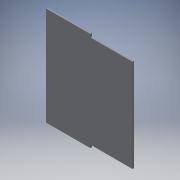
# Autodesk Inventor part: Dach2
Saved by Autodesk Inventor 2019 (Build 230136000, 136)
## iProperties
Created: 2023-01-16
Part Number: Dach2
Material: Ogólny
Document SubType Name: Modeling
Designer: Michał
Density: 1 g/cm^3
Appearance: Domyślna
Author: Michał
Autodesk Inventor part; units mm, degrees
ref_plane "YZ Plane" through (0, 0, 0) normal (1, 0, 0) x (0, 1, 0)
ref_plane "XZ Plane" through (0, 0, 0) normal (0, 1, 0) x (-1, 0, 0)
ref_plane "XY Plane" through (0, 0, 0) normal (0, 0, 1) x (1, 0, 0)
sketch "Szkic1" plane through (0, 0, 0) normal (0, 0, 1) x (1, 0, 0)
  line L0 (-30.3153, -10.76) -> (-97.6449, -10.76) construction
  line L1 (-30.3153, -10.76) -> (-97.6449, -10.76) construction
  line L2 (-101.109, 124.5875) -> (-101.109, -11.5875) construction
  line L3 (-30.3153, 123.76) -> (-97.6449, 123.76) construction
  line L4 (16.507, 124.589) -> (16.507, -11.589) construction
  line L5 (-40.75, -6.5) -> (16.507, -6.5) construction
  line L6 (-40.75, 119.5) -> (16.507, 119.5) construction
  line L7 (-100.909, 123.56) -> (-40.75, 123.56)
  line L8 (-40.75, 123.56) -> (-40.75, -10.56)
  line L9 (-40.75, -10.56) -> (-100.909, -10.56)
  line L10 (-100.909, -10.56) -> (-100.909, 123.56)
  line L11 (-40.75, 119.5) -> (16.307, 119.5)
  line L12 (16.307, 119.5) -> (16.307, -6.5)
  line L13 (16.307, -6.5) -> (-40.75, -6.5)
  line L14 (-40.75, -6.5) -> (-40.75, 119.5)
  line L15 (-100.909, 56.5) -> (-101.109, 56.5) construction
  line L16 (16.307, 56.5) -> (16.507, 56.5) construction
  line L17 (-70.8295, -10.56) -> (-70.8295, -10.76) construction
  line L18 (-70.8295, 123.56) -> (-70.8295, 123.76) construction
  line L19 (-89.609, 108.26) -> (-100.609, 108.26)
  line L20 (-89.609, 115.26) -> (-89.609, 108.26)
  line L21 (-100.609, 115.26) -> (-89.609, 115.26)
  line L22 (-100.609, 108.26) -> (-100.609, 115.26)
  line L23 (-100.609, 115.26) -> (-100.909, 115.26)
  line L24 (-100.609, 108.26) -> (-100.909, 108.26)
  line L25 (-87.109, 6.24) -> (-99.109, 6.24) projected
  line L26 (-99.109, -2.76) -> (-99.109, 6.24) projected
  line L27 (-87.109, -2.76) -> (-99.109, -2.76) projected
  line L28 (-87.109, 6.24) -> (-87.109, -2.76) projected
  line L29 (-75.109, 13.24) -> (-75.109, 6.24)
  line L30 (-75.109, 6.24) -> (-86.109, 6.24)
  line L31 (-86.109, 6.24) -> (-86.109, 13.24)
  line L32 (-86.109, 13.24) -> (-75.109, 13.24)
  line L33 (-85.609, 5.24) -> (-75.109, 5.24)
  line L34 (-75.109, 5.24) -> (-75.109, -9.76)
  line L35 (-75.109, -9.76) -> (-85.609, -9.76)
  line L36 (-85.609, -9.76) -> (-85.609, 5.24)
  line L37 (-76.109, -9.06) -> (-84.609, -9.06) construction
  line L38 (-84.609, -9.06) -> (-84.609, 4.54) construction
  line L39 (-84.609, 4.54) -> (-76.109, 4.54) construction
  line L40 (-76.109, 4.54) -> (-76.109, -9.06) construction
  line L41 (-75.109, 5.24) -> (-75.109, -9.76) construction
  line L42 (-85.609, 5.24) -> (-75.109, 5.24) construction
  line L43 (-85.609, -9.76) -> (-85.609, 5.24) construction
  line L44 (-75.109, -9.76) -> (-85.609, -9.76) construction
  line L45 (-75.109, -2.26) -> (-75.109, -2.26) construction
  line L46 (-75.109, -9.76) -> (-85.609, -9.76)
  line L47 (-85.609, -9.76) -> (-85.609, -10.56)
  line L48 (-85.609, -10.56) -> (-75.109, -10.56)
  line L49 (-75.109, -10.56) -> (-75.109, -9.76)
  point P0 (0, 0)
  point P1 (-40.75, 56.5)
  dimension "d0" = 0.2
  constraints: 62 end point, 10 midpoint, 10 perpendicular, 8 horizontal, 8 parallel, 7 collinear, 7 point on line, 4 vertical, 2 equal length, 8 other
  measures "d0" distance between parallel lines of L4 L12
ref_plane "Płaszczyzna konstrukcyjna1" through (16.507, -11.589, 2) normal (0, 0, 1) x (1, 0, 0)
extrude "Wyciągnięcie proste3" add sketch "Szkic1" along normal blind 2 contours L7 L8 L9 L49 L34 L33 L36 L47 L10 L24 L19 L20 L21 L23 | L11 L12 L13 L8
sketch "Szkic2" plane through (-100.909, 123.56, 2) normal (0, 0, 1) x (1, 0, 0)
  line L0 (98.216, -22.2759) -> (98.216, -111.8441) construction
  line L1 (98.216, -111.8441) -> (83.8317, -111.8441) construction
  line L2 (83.8317, -111.8441) -> (83.8317, -22.2759) construction
  line L3 (83.8317, -22.2759) -> (98.216, -22.2759) construction
  line L4 (81.8317, -22.2759) -> (81.8317, -80.9218) construction
  line L5 (81.8317, -80.9218) -> (73.6071, -80.9218) construction
  line L6 (73.6071, -80.9218) -> (73.6071, -22.2759) construction
  line L7 (73.6071, -22.2759) -> (81.8317, -22.2759) construction
  line L8 (35.5742, -109.2952) -> (35.5742, -118.3334) construction
  line L9 (35.5742, -118.3334) -> (29.6072, -118.3334) construction
  line L10 (29.6072, -118.3334) -> (29.6072, -109.2952) construction
  line L11 (29.6072, -109.2952) -> (35.5742, -109.2952) construction
  line L12 (36.1418, -121.3134) -> (36.1418, -131.569) construction
  line L13 (36.1418, -131.569) -> (29.1418, -131.569) construction
  line L14 (29.1418, -131.569) -> (29.1418, -121.3134) construction
  line L15 (29.1418, -121.3134) -> (36.1418, -121.3134) construction
  line L16 (21.349, -9.0957) -> (21.349, -16.2294) construction
  line L17 (21.349, -16.2294) -> (14.3259, -16.2294) construction
  line L18 (14.3259, -16.2294) -> (14.3259, -9.0957) construction
  line L19 (14.3259, -9.0957) -> (21.349, -9.0957) construction
  line L20 (13.8, -117.32) -> (13.8, -126.32) construction
  line L21 (13.8, -126.32) -> (1.8, -126.32) construction
  line L22 (1.8, -126.32) -> (1.8, -117.32) construction
  line L23 (1.8, -117.32) -> (13.8, -117.32) construction
  line L24 (25.8, -117.32) -> (14.8, -117.32) construction
  line L25 (14.8, -117.32) -> (14.8, -110.32) construction
  line L26 (14.8, -110.32) -> (25.8, -110.32) construction
  line L27 (25.8, -110.32) -> (25.8, -117.32) construction
  line L28 (60.159, -130.06) -> (117.216, -130.06) construction
  line L29 (117.216, -130.06) -> (117.216, -4.06) construction
  line L30 (117.216, -4.06) -> (60.159, -4.06) construction
  line L31 (60.159, -4.06) -> (60.159, 0) construction
  line L32 (60.159, 0) -> (0, 0) construction
  line L33 (0, 0) -> (0, -8.3) construction
  line L34 (0, -8.3) -> (11.3, -8.3) construction
  line L35 (11.3, -8.3) -> (11.3, -15.3) construction
  line L36 (11.3, -15.3) -> (0, -15.3) construction
  line L37 (0, -15.3) -> (0, -134.12) construction
  line L38 (25.8, -134.12) -> (60.159, -134.12) construction
  line L39 (60.159, -134.12) -> (60.159, -130.06) construction
  line L40 (25.8, -118.32) -> (25.8, -134.12) projected
  line L41 (0, -134.12) -> (15.3, -134.12) projected
  line L42 (15.3, -134.12) -> (15.3, -118.32) projected
  line L43 (15.3, -118.32) -> (25.8, -118.32) projected
  line L44 (60.159, -12.06) -> (60.159, -27.262)
  line L45 (60.159, -27.262) -> (51.696, -27.262)
  line L46 (60.159, -12.06) -> (57.525, -12.06)
  line L47 (57.525, -12.06) -> (57.525, -24.629)
  line L48 (57.525, -24.629) -> (54.333, -24.629)
  line L49 (54.333, -24.629) -> (54.333, -12.06)
  line L50 (54.333, -12.06) -> (48.639, -12.06)
  line L51 (48.639, -12.06) -> (48.639, -14.694)
  line L52 (48.639, -14.694) -> (51.696, -14.694)
  line L53 (51.696, -14.694) -> (51.696, -27.262)
  line L54 (60.159, -27.262) -> (60.159, -30.569)
  line L55 (60.159, -30.569) -> (48.639, -30.569)
  line L56 (48.639, -30.569) -> (48.639, -33.203)
  line L57 (48.639, -33.203) -> (57.525, -33.203)
  line L58 (57.525, -33.203) -> (57.525, -44.265)
  line L59 (57.525, -44.265) -> (48.639, -44.265)
  line L60 (48.639, -44.265) -> (48.639, -46.899)
  line L61 (48.639, -46.899) -> (60.159, -46.899)
  line L62 (60.159, -46.899) -> (60.159, -30.569)
  line L63 (57.525, -33.203) -> (57.525, -37.419)
  line L64 (57.525, -44.265) -> (57.525, -40.049)
  line L65 (55.972, -40.051) -> (55.972, -37.417)
  line L66 (55.972, -37.417) -> (48.639, -37.417)
  line L67 (48.639, -37.417) -> (48.639, -40.051)
  line L68 (48.639, -40.051) -> (55.972, -40.051)
  line L69 (48.639, -33.203) -> (48.639, -37.417) construction
  line L70 (48.639, -40.051) -> (48.639, -44.265) construction
  line L71 (60.159, -4.06) -> (60.159, 0) construction
  line L72 (80.001, -29.88) -> (77.8613, -28.2983)
  line L73 (77.8613, -28.2983) -> (77.8613, -24.0836)
  line L74 (77.8613, -24.0836) -> (75.8646, -24.0836)
  line L75 (75.8646, -24.0836) -> (74.8317, -22.2805)
  line L76 (74.8317, -22.2805) -> (81.8317, -22.2805)
  line L77 (81.8317, -22.2805) -> (81.8317, -28.5197)
  line L78 (81.8317, -28.5197) -> (80.001, -29.88)
  line L79 (79.8765, -28.0216) -> (80.5036, -27.5467)
  line L80 (80.5036, -27.5467) -> (80.5036, -24.0836)
  line L81 (80.5036, -24.0836) -> (79.2171, -24.0836)
  line L82 (79.2171, -24.0836) -> (79.2171, -27.5467)
  line L83 (79.2171, -27.5467) -> (79.8765, -28.0216)
  line L84 (75.8554, -32.2733) -> (74.8317, -30.4702)
  line L85 (74.8317, -30.4702) -> (81.8317, -30.4702)
  line L86 (81.8317, -30.4702) -> (81.8317, -32.2733)
  line L87 (81.8317, -32.2733) -> (75.8554, -32.2733)
  line L88 (75.8646, -40.8965) -> (75.8646, -39.0934)
  line L89 (75.8646, -39.0934) -> (77.3264, -39.0934)
  line L90 (77.3264, -39.0934) -> (77.8613, -38.5447)
  line L91 (77.8613, -38.5447) -> (77.8613, -35.1)
  line L92 (77.8613, -35.1) -> (75.8646, -35.1)
  line L93 (75.8646, -35.1) -> (74.8317, -33.297)
  line L94 (74.8317, -33.297) -> (81.8317, -33.297)
  line L95 (81.8317, -33.297) -> (81.8317, -39.5361)
  line L96 (81.8317, -39.5361) -> (80.001, -40.8965)
  line L97 (80.001, -40.8965) -> (78.613, -39.8635)
  line L98 (78.613, -39.8635) -> (77.5754, -40.8965)
  line L99 (77.5754, -40.8965) -> (75.8646, -40.8965)
  line L100 (79.8765, -39.0427) -> (80.5036, -38.5631)
  line L101 (80.5036, -38.5631) -> (80.5036, -35.1)
  line L102 (80.5036, -35.1) -> (79.2171, -35.1)
  line L103 (79.2171, -35.1) -> (79.2171, -38.5585)
  line L104 (79.2171, -38.5585) -> (79.8765, -39.0427)
  line L105 (75.8554, -49.1646) -> (75.8554, -47.3523)
  line L106 (75.8554, -47.3523) -> (77.5754, -47.3523)
  line L107 (77.5754, -47.3523) -> (77.5754, -43.7232)
  line L108 (77.5754, -43.7232) -> (75.8554, -43.7232)
  line L109 (75.8554, -43.7232) -> (74.8317, -41.9202)
  line L110 (74.8317, -41.9202) -> (80.4944, -41.9202)
  line L111 (80.4944, -41.9202) -> (81.8317, -43.2759)
  line L112 (81.8317, -43.2759) -> (81.8317, -47.8088)
  line L113 (81.8317, -47.8088) -> (80.4944, -49.1646)
  line L114 (80.4944, -49.1646) -> (75.8554, -49.1646)
  line L115 (78.8943, -47.3523) -> (80.4944, -47.3523)
  line L116 (80.4944, -47.3523) -> (80.4944, -43.7232)
  line L117 (80.4944, -43.7232) -> (78.8943, -43.7232)
  line L118 (78.8943, -43.7232) -> (78.8943, -47.3523)
  line L119 (75.8646, -59.4478) -> (75.8646, -57.6448)
  line L120 (75.8646, -57.6448) -> (79.6828, -57.6448)
  line L121 (79.6828, -57.6448) -> (76.6071, -55.4037)
  line L122 (76.6071, -55.4037) -> (76.6071, -54.237)
  line L123 (76.6071, -54.237) -> (79.6828, -52.0098)
  line L124 (79.6828, -52.0098) -> (75.8646, -52.0098)
  line L125 (75.8646, -52.0098) -> (74.8317, -50.2067)
  line L126 (74.8317, -50.2067) -> (81.8317, -50.2067)
  line L127 (81.8317, -50.2067) -> (81.8317, -52.245)
  line L128 (81.8317, -52.245) -> (78.281, -54.8273)
  line L129 (78.281, -54.8273) -> (81.8317, -57.4004)
  line L130 (81.8317, -57.4004) -> (81.8317, -59.4478)
  line L131 (81.8317, -59.4478) -> (75.8646, -59.4478)
  line L132 (75.8554, -62.2654) -> (74.8317, -60.4623)
  line L133 (74.8317, -60.4623) -> (81.8317, -60.4623)
  line L134 (81.8317, -60.4623) -> (81.8317, -62.2654)
  line L135 (81.8317, -62.2654) -> (75.8554, -62.2654)
  line L136 (78.8436, -70.967) -> (75.8554, -69.2746)
  line L137 (75.8554, -69.2746) -> (75.8554, -63.2891)
  line L138 (75.8554, -63.2891) -> (81.8317, -63.2891)
  line L139 (81.8317, -63.2891) -> (81.8317, -69.2746)
  line L140 (81.8317, -69.2746) -> (78.8436, -70.967)
  line L141 (78.8482, -69.0164) -> (80.4944, -68.0849)
  line L142 (80.4944, -68.0849) -> (80.4944, -65.0921)
  line L143 (80.4944, -65.0921) -> (77.1927, -65.0921)
  line L144 (77.1927, -65.0921) -> (77.1927, -68.0803)
  line L145 (77.1927, -68.0803) -> (78.8482, -69.0164)
  line L146 (75.8554, -79.0737) -> (75.8554, -77.2614)
  line L147 (75.8554, -77.2614) -> (77.5754, -77.2614)
  line L148 (77.5754, -77.2614) -> (77.5754, -73.6323)
  line L149 (77.5754, -73.6323) -> (75.8554, -73.6323)
  line L150 (75.8554, -73.6323) -> (74.8317, -71.8293)
  line L151 (74.8317, -71.8293) -> (80.4944, -71.8293)
  line L152 (80.4944, -71.8293) -> (81.8317, -73.185)
  line L153 (81.8317, -73.185) -> (81.8317, -77.7179)
  line L154 (81.8317, -77.7179) -> (80.4944, -79.0737)
  line L155 (80.4944, -79.0737) -> (75.8554, -79.0737)
  line L156 (78.8943, -77.2614) -> (80.4944, -77.2614)
  line L157 (80.4944, -77.2614) -> (80.4944, -73.6323)
  line L158 (80.4944, -73.6323) -> (78.8943, -73.6323)
  line L159 (78.8943, -73.6323) -> (78.8943, -77.2614)
  line L160 (86.1923, -35.3115) -> (86.1923, -32.2206)
  line L161 (86.1923, -32.2206) -> (88.6982, -32.2206)
  line L162 (88.6982, -32.2206) -> (89.6152, -31.2799)
  line L163 (89.6152, -31.2799) -> (89.6152, -25.3747)
  line L164 (89.6152, -25.3747) -> (86.1923, -25.3747)
  line L165 (86.1923, -25.3747) -> (84.4215, -22.2838)
  line L166 (84.4215, -22.2838) -> (96.4215, -22.2838)
  line L167 (96.4215, -22.2838) -> (96.4215, -32.9795)
  line L168 (96.4215, -32.9795) -> (93.2832, -35.3115)
  line L169 (93.2832, -35.3115) -> (90.9037, -33.5407)
  line L170 (90.9037, -33.5407) -> (89.1251, -35.3115)
  line L171 (89.1251, -35.3115) -> (86.1923, -35.3115)
  line L172 (93.0697, -32.1336) -> (94.1448, -31.3115)
  line L173 (94.1448, -31.3115) -> (94.1448, -25.3747)
  line L174 (94.1448, -25.3747) -> (91.9393, -25.3747)
  line L175 (91.9393, -25.3747) -> (91.9393, -31.3036)
  line L176 (91.9393, -31.3036) -> (93.0697, -32.1336)
  line L177 (88.5164, -50.2522) -> (86.1923, -47.9281)
  line L178 (86.1923, -47.9281) -> (86.1923, -39.3905)
  line L179 (86.1923, -39.3905) -> (88.5164, -37.0664)
  line L180 (88.5164, -37.0664) -> (94.0974, -37.0664)
  line L181 (94.0974, -37.0664) -> (96.4215, -39.3905)
  line L182 (96.4215, -39.3905) -> (96.4215, -47.9281)
  line L183 (96.4215, -47.9281) -> (94.0974, -50.2522)
  line L184 (94.0974, -50.2522) -> (88.5164, -50.2522)
  line L185 (88.4689, -47.1613) -> (94.1448, -47.1613)
  line L186 (94.1448, -47.1613) -> (94.1448, -40.1573)
  line L187 (94.1448, -40.1573) -> (88.4689, -40.1573)
  line L188 (88.4689, -40.1573) -> (88.4689, -47.1613)
  line L189 (89.3227, -65.0664) -> (86.1765, -62.7423)
  line L190 (86.1765, -62.7423) -> (86.1765, -51.9044)
  line L191 (86.1765, -51.9044) -> (96.4215, -51.9044)
  line L192 (96.4215, -51.9044) -> (96.4215, -62.7423)
  line L193 (96.4215, -62.7423) -> (93.2753, -65.0664)
  line L194 (93.2753, -65.0664) -> (91.299, -63.6119)
  line L195 (91.299, -63.6119) -> (89.3227, -65.0664)
  line L196 (89.3227, -61.683) -> (90.2555, -60.932)
  line L197 (90.2555, -60.932) -> (90.2555, -54.9953)
  line L198 (90.2555, -54.9953) -> (88.4689, -54.9953)
  line L199 (88.4689, -54.9953) -> (88.4689, -60.932)
  line L200 (88.4689, -60.932) -> (89.3227, -61.683)
  line L201 (93.2753, -61.683) -> (94.129, -60.932)
  line L202 (94.129, -60.932) -> (94.129, -54.9953)
  line L203 (94.129, -54.9953) -> (92.3425, -54.9953)
  line L204 (92.3425, -54.9953) -> (92.3425, -60.932)
  line L205 (92.3425, -60.932) -> (93.2753, -61.683)
  line L206 (88.5164, -79.8728) -> (86.1923, -77.5486)
  line L207 (86.1923, -77.5486) -> (86.1923, -69.0111)
  line L208 (86.1923, -69.0111) -> (88.5164, -66.687)
  line L209 (88.5164, -66.687) -> (94.0974, -66.687)
  line L210 (94.0974, -66.687) -> (96.4215, -69.0111)
  line L211 (96.4215, -69.0111) -> (96.4215, -77.5486)
  line L212 (96.4215, -77.5486) -> (94.0974, -79.8728)
  line L213 (94.0974, -79.8728) -> (88.5164, -79.8728)
  line L214 (88.4689, -76.7818) -> (94.1448, -76.7818)
  line L215 (94.1448, -76.7818) -> (94.1448, -69.7779)
  line L216 (94.1448, -69.7779) -> (88.4689, -69.7779)
  line L217 (88.4689, -69.7779) -> (88.4689, -76.7818)
  line L218 (86.1765, -84.6158) -> (84.4215, -81.5249)
  line L219 (84.4215, -81.5249) -> (96.4215, -81.5249)
  line L220 (96.4215, -81.5249) -> (96.4215, -84.6158)
  line L221 (96.4215, -84.6158) -> (86.1765, -84.6158)
  line L222 (88.4689, -98.2522) -> (86.1765, -95.9597)
  line L223 (86.1765, -95.9597) -> (86.1765, -86.3708)
  line L224 (86.1765, -86.3708) -> (96.4294, -86.3708)
  line L225 (96.4294, -86.3708) -> (98.216, -89.4617)
  line L226 (98.216, -89.4617) -> (88.4689, -89.4617)
  line L227 (88.4689, -89.4617) -> (88.4689, -98.2522)
  line L228 (88.5164, -111.7858) -> (86.1923, -109.4617)
  line L229 (86.1923, -109.4617) -> (86.1923, -100.9241)
  line L230 (86.1923, -100.9241) -> (88.5164, -98.6)
  line L231 (88.5164, -98.6) -> (94.0974, -98.6)
  line L232 (94.0974, -98.6) -> (96.4215, -100.9241)
  line L233 (96.4215, -100.9241) -> (96.4215, -109.4617)
  line L234 (96.4215, -109.4617) -> (94.0974, -111.7858)
  line L235 (94.0974, -111.7858) -> (88.5164, -111.7858)
  line L236 (88.4689, -108.6949) -> (94.1448, -108.6949)
  line L237 (94.1448, -108.6949) -> (94.1448, -101.6909)
  line L238 (94.1448, -101.6909) -> (88.4689, -101.6909)
  line L239 (88.4689, -101.6909) -> (88.4689, -108.6949)
  line L240 (30.1748, -130.5591) -> (30.1748, -128.7561)
  line L241 (30.1748, -128.7561) -> (33.9929, -128.7561)
  line L242 (33.9929, -128.7561) -> (30.9172, -126.515)
  line L243 (30.9172, -126.515) -> (30.9172, -125.3483)
  line L244 (30.9172, -125.3483) -> (33.9929, -123.121)
  line L245 (33.9929, -123.121) -> (30.1748, -123.121)
  line L246 (30.1748, -123.121) -> (29.1418, -121.318)
  line L247 (29.1418, -121.318) -> (36.1418, -121.318)
  line L248 (36.1418, -121.318) -> (36.1418, -123.3562)
  line L249 (36.1418, -123.3562) -> (32.5911, -125.9385)
  line L250 (32.5911, -125.9385) -> (36.1418, -128.5117)
  line L251 (36.1418, -128.5117) -> (36.1418, -130.5591)
  line L252 (36.1418, -130.5591) -> (30.1748, -130.5591)
  line L253 (31.4425, -117.5864) -> (29.6072, -116.2307)
  line L254 (29.6072, -116.2307) -> (29.6072, -109.2998)
  line L255 (29.6072, -109.2998) -> (30.9352, -110.6279)
  line L256 (30.9352, -110.6279) -> (30.9352, -115.1747)
  line L257 (30.9352, -115.1747) -> (31.4425, -115.5989)
  line L258 (31.4425, -115.5989) -> (31.9774, -115.1793)
  line L259 (31.9774, -115.1793) -> (31.9774, -110.6187)
  line L260 (31.9774, -110.6187) -> (33.7389, -109.2998)
  line L261 (33.7389, -109.2998) -> (35.5742, -110.6556)
  line L262 (35.5742, -110.6556) -> (35.5742, -117.5864)
  line L263 (35.5742, -117.5864) -> (34.2462, -116.2491)
  line L264 (34.2462, -116.2491) -> (34.2462, -111.7116)
  line L265 (34.2462, -111.7116) -> (33.7389, -111.2735)
  line L266 (33.7389, -111.2735) -> (33.204, -111.7116)
  line L267 (33.204, -111.7116) -> (33.204, -116.2722)
  line L268 (33.204, -116.2722) -> (31.4425, -117.5864)
  line L269 (15.6632, -16.0311) -> (14.3259, -14.6939)
  line L270 (14.3259, -14.6939) -> (14.3259, -9.1003)
  line L271 (14.3259, -9.1003) -> (20.3068, -9.1003)
  line L272 (20.3068, -9.1003) -> (21.349, -10.9033)
  line L273 (21.349, -10.9033) -> (15.6632, -10.9033)
  line L274 (15.6632, -10.9033) -> (15.6632, -16.0311)
  point P0 (98.216, -67.06)
  point P1 (117.216, -67.06)
  dimension "d3" = 2
  dimension "d11" = 15.202
  dimension "d12" = 8.463
  dimension "d14" = 12.569
  dimension "d15" = 3.192
  dimension "d16" = 5.694
  dimension "d18" = 3.307
  dimension "d19" = 2.634
  dimension "d20" = 8.886
  dimension "d21" = 11.062
  dimension "d23" = 4.216
  dimension "d24" = 4.216
  dimension "d26" = 1.553
  dimension "d27" = 8
  constraints: 54 end point, 14 perpendicular, 7 collinear, 7 point on line, 5 equal length, 3 parallel, 2 midpoint, 1 horizontal alignment, 10 other
  measures "d3" distance between parallel lines of L2 L4
  measures "d11" distance of L44.start L45.start
  measures "d12" distance of L45.start L45.end
  measures "d14" distance of L46.end L47.end
  measures "d15" distance of L47.end L48.end
  measures "d16" distance of L49.end L50.end
  measures "d18" distance of L45.start L62.end
  measures "d19" distance of L55.end L57.start
  measures "d20" distance of L57.start L58.start
  measures "d21" distance of L58.start L64.start
  measures "d23" distance of L58.start L63.end
  measures "d24" distance of L64.start L64.end
  measures "d26" distance between parallel lines of L65 L58
  measures "d27" distance of L30.end L44.start
extrude "Wyciągnięcie proste2" cut sketch "Szkic2" against normal blind 1
